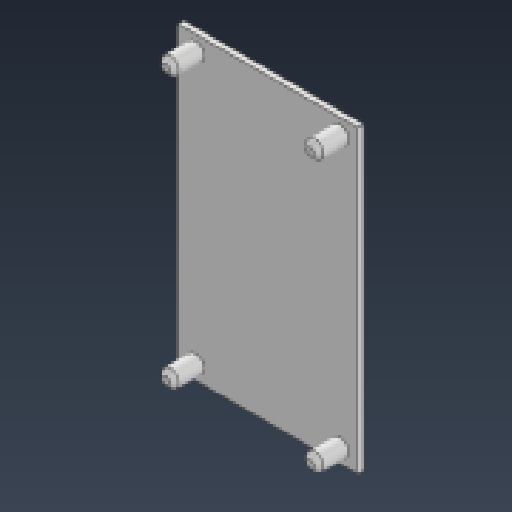
# Autodesk Inventor part: buck_holes_check
Saved by Autodesk Inventor 2023 (Build 270158000, 158)
## iProperties
Created: 2025-12-26
Part Number: buck_holes_check
Material: Generic
Document SubType Name: Modeling
Designer: szymo
Density: 1 g/cm^3
Appearance: Default
Author: szymo
Autodesk Inventor part; units mm, degrees
ref_plane "YZ Plane" through (0, 0, 0) normal (1, 0, 0) x (0, 1, 0)
ref_plane "XZ Plane" through (0, 0, 0) normal (0, 1, 0) x (-1, 0, 0)
ref_plane "XY Plane" through (0, 0, 0) normal (0, 0, 1) x (1, 0, 0)
sketch "Sketch1" plane through (0, 0, 0) normal (0, 0, 1) x (1, 0, 0)
  circle A0 centre (12.05, 22.55) radius 1.45 projected
  circle A1 centre (-12.05, 22.55) radius 1.45 projected
  circle A2 centre (-12.05, -22.55) radius 1.45 projected
  circle A3 centre (12.05, -22.55) radius 1.45 projected
  line L0 (15, -25) -> (-15, -25) projected
  line L1 (15, 25) -> (15, -25) projected
  line L2 (-15, 25) -> (15, 25) projected
  line L3 (-15, -25) -> (-15, 25) projected
  point P0 (0, 0)
extrude "Extrusion1" add sketch "Sketch1" along normal blind 1
sketch "Sketch2" plane through (0, 0, 1) normal (0, 0, 1) x (1, 0, 0)
  line L0 (15, 25) -> (-15, 25) projected
  line L1 (-15, 25) -> (-15, -25) projected
  line L2 (-15, -25) -> (15, -25) projected
  line L3 (15, -25) -> (15, 25) projected
  circle A0 centre (12.05, -22.55) radius 1.45 projected
  circle A1 centre (-12.05, -22.55) radius 1.45 projected
  circle A2 centre (-12.05, 22.55) radius 1.45 projected
  circle A3 centre (12.05, 22.55) radius 1.45 projected
  point P0 (0, 0)
extrude "Extrusion2" add sketch "Sketch2" along normal blind 5 and the other way blind 1 contours A0 | A1 | A2 | A3
chamfer "Chamfer1" distance 0.8 angle 45 4 edges at (-13.5, -22.55, 6) (-13.5, 22.55, 6) (10.6, 22.55, 6) (10.6, -22.55, 6)
body "Solid1"
